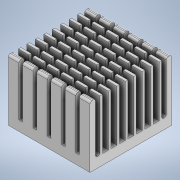
# Autodesk Inventor part: Część2
Saved by Autodesk Inventor 2022 (Build 260153000, 153)
## iProperties
Created: 2022-09-09
Part Number: Część2
Material: Ogólny
Document SubType Name: Modeling
Designer: kosak
Density: 1 g/cm^3
Appearance: Domyślna
Author: kosak
Autodesk Inventor part; units mm, degrees
ref_plane "YZ Plane" through (0, 0, 0) normal (1, 0, 0) x (0, 1, 0)
ref_plane "XZ Plane" through (0, 0, 0) normal (0, 1, 0) x (-1, 0, 0)
ref_plane "XY Plane" through (0, 0, 0) normal (0, 0, 1) x (1, 0, 0)
sketch "Szkic1" plane through (0, 0, 0) normal (0, 1, 0) x (-1, 0, 0)
  line L0 (0, 0) -> (40, 0)
  line L1 (40, 0) -> (40, -40)
  line L2 (40, -40) -> (0, -40)
  line L3 (0, -40) -> (0, 0)
  dimension "d0" = 40
  dimension "d1" = 40
  constraints: 8 end point, 2 parallel, 1 horizontal, 1 perpendicular
  measures "d0" distance of L1.end L2.end
  measures "d1" distance of L0.end L1.end
extrude "Wyciągnięcie proste1" add sketch "Szkic1" along normal blind 5
sketch "Szkic2" plane through (0, 5, 0) normal (0, 1, 0) x (1, 0, 0)
  line L0 (0, 20) -> (-40, 20)
  line L1 (-20, 0) -> (-20, 40)
  line L2 (0, 40) -> (-5.2, 40)
  line L3 (-5.2, 40) -> (-5.2, 37.35)
  line L4 (-5.2, 37.35) -> (0, 37.35)
  line L5 (0, 37.35) -> (0, 40)
  line L6 (-40, 37.35) -> (-40, 40)
  line L7 (-34.8, 37.35) -> (-40, 37.35)
  line L8 (-34.8, 40) -> (-34.8, 37.35)
  line L9 (-40, 40) -> (-34.8, 40)
  line L10 (-12.16, 40) -> (-12.16, 37.35)
  line L11 (-6.96, 40) -> (-12.16, 40)
  line L12 (-12.16, 37.35) -> (-6.96, 37.35)
  line L13 (-6.96, 37.35) -> (-6.96, 40)
  line L14 (-19.12, 40) -> (-19.12, 37.35)
  line L15 (-13.92, 40) -> (-19.12, 40)
  line L16 (-19.12, 37.35) -> (-13.92, 37.35)
  line L17 (-13.92, 37.35) -> (-13.92, 40)
  line L18 (-26.08, 40) -> (-26.08, 37.35)
  line L19 (-20.88, 40) -> (-26.08, 40)
  line L20 (-26.08, 37.35) -> (-20.88, 37.35)
  line L21 (-20.88, 37.35) -> (-20.88, 40)
  line L22 (-33.04, 40) -> (-33.04, 37.35)
  line L23 (-27.84, 40) -> (-33.04, 40)
  line L24 (-33.04, 37.35) -> (-27.84, 37.35)
  line L25 (-27.84, 37.35) -> (-27.84, 40)
  line L26 (-40, 40) -> (-40, 37.35)
  line L27 (-34.8, 40) -> (-40, 40)
  line L28 (-40, 37.35) -> (-34.8, 37.35)
  line L29 (-34.8, 37.35) -> (-34.8, 40)
  line L30 (-34.8, 2.65) -> (-40, 2.65)
  line L31 (-40, 2.65) -> (-40, 0)
  line L32 (-40, 0) -> (-34.8, 0)
  line L33 (-5.2, 0) -> (-5.2, 2.65)
  line L34 (-5.2, 2.65) -> (0, 2.65)
  line L35 (0, 2.65) -> (0, 0)
  line L36 (0, 0) -> (-5.2, 0)
  line L37 (-12.16, 0) -> (-12.16, 2.65)
  line L38 (-6.96, 0) -> (-12.16, 0)
  line L39 (-12.16, 2.65) -> (-6.96, 2.65)
  line L40 (-6.96, 2.65) -> (-6.96, 0)
  line L41 (-19.12, 0) -> (-19.12, 2.65)
  line L42 (-13.92, 0) -> (-19.12, 0)
  line L43 (-19.12, 2.65) -> (-13.92, 2.65)
  line L44 (-13.92, 2.65) -> (-13.92, 0)
  line L45 (-26.08, 0) -> (-26.08, 2.65)
  line L46 (-20.88, 0) -> (-26.08, 0)
  line L47 (-26.08, 2.65) -> (-20.88, 2.65)
  line L48 (-20.88, 2.65) -> (-20.88, 0)
  line L49 (-33.04, 0) -> (-33.04, 2.65)
  line L50 (-27.84, 0) -> (-33.04, 0)
  line L51 (-33.04, 2.65) -> (-27.84, 2.65)
  line L52 (-27.84, 2.65) -> (-27.84, 0)
  line L53 (-34.8, 2.65) -> (-34.8, 0)
  line L54 (-2.6, 37.35) -> (-2.6, 35.1)
  line L55 (0, 0) -> (0, 40) projected
  line L56 (0, 35.1) -> (-5.2, 35.1)
  line L57 (-5.2, 35.1) -> (-5.2, 33.86)
  line L58 (-5.2, 33.86) -> (0, 33.86)
  line L59 (0, 33.86) -> (0, 35.1)
  line L60 (-6.96, 35.1) -> (-12.16, 35.1)
  line L61 (-12.16, 33.86) -> (-6.96, 33.86)
  line L62 (-12.16, 35.1) -> (-12.16, 33.86)
  line L63 (-6.96, 33.86) -> (-6.96, 35.1)
  line L64 (-13.92, 35.1) -> (-19.12, 35.1)
  line L65 (-19.12, 33.86) -> (-13.92, 33.86)
  line L66 (-19.12, 35.1) -> (-19.12, 33.86)
  line L67 (-13.92, 33.86) -> (-13.92, 35.1)
  line L68 (-20.88, 35.1) -> (-26.08, 35.1)
  line L69 (-26.08, 33.86) -> (-20.88, 33.86)
  line L70 (-26.08, 35.1) -> (-26.08, 33.86)
  line L71 (-20.88, 33.86) -> (-20.88, 35.1)
  line L72 (-27.84, 35.1) -> (-33.04, 35.1)
  line L73 (-33.04, 33.86) -> (-27.84, 33.86)
  line L74 (-33.04, 35.1) -> (-33.04, 33.86)
  line L75 (-27.84, 33.86) -> (-27.84, 35.1)
  line L76 (-34.8, 35.1) -> (-40, 35.1)
  line L77 (-40, 33.86) -> (-34.8, 33.86)
  line L78 (-40, 35.1) -> (-40, 33.86)
  line L79 (-34.8, 33.86) -> (-34.8, 35.1)
  line L80 (0, 4.9) -> (-5.2, 4.9)
  line L81 (-5.2, 4.9) -> (-5.2, 6.14)
  line L82 (-5.2, 6.14) -> (0, 6.14)
  line L83 (0, 30.963) -> (-5.2, 30.963)
  line L84 (-5.2, 29.723) -> (0, 29.723)
  line L85 (-5.2, 30.963) -> (-5.2, 29.723)
  line L86 (0, 29.723) -> (0, 30.963)
  line L87 (0, 26.826) -> (-5.2, 26.826)
  line L88 (-5.2, 25.586) -> (0, 25.586)
  line L89 (-5.2, 26.826) -> (-5.2, 25.586)
  line L90 (0, 25.586) -> (0, 26.826)
  line L91 (0, 22.689) -> (-5.2, 22.689)
  line L92 (-5.2, 21.449) -> (0, 21.449)
  line L93 (-5.2, 22.689) -> (-5.2, 21.449)
  line L94 (0, 21.449) -> (0, 22.689)
  line L95 (0, 18.552) -> (-5.2, 18.552)
  line L96 (-5.2, 17.312) -> (0, 17.312)
  line L97 (-5.2, 18.552) -> (-5.2, 17.312)
  line L98 (0, 17.312) -> (0, 18.552)
  line L99 (0, 14.415) -> (-5.2, 14.415)
  line L100 (-5.2, 13.175) -> (0, 13.175)
  line L101 (-5.2, 14.415) -> (-5.2, 13.175)
  line L102 (0, 13.175) -> (0, 14.415)
  line L103 (0, 10.278) -> (-5.2, 10.278)
  line L104 (-5.2, 9.038) -> (0, 9.038)
  line L105 (-5.2, 10.278) -> (-5.2, 9.038)
  line L106 (0, 9.038) -> (0, 10.278)
  line L107 (0, 6.141) -> (-5.2, 6.141)
  line L108 (-5.2, 4.901) -> (0, 4.901)
  line L109 (-5.2, 6.141) -> (-5.2, 4.901)
  line L110 (0, 4.901) -> (0, 6.141)
  line L111 (-6.96, 30.963) -> (-12.16, 30.963)
  line L112 (-6.96, 29.723) -> (-6.96, 30.963)
  line L113 (-12.16, 29.723) -> (-6.96, 29.723)
  line L114 (-12.16, 30.963) -> (-12.16, 29.723)
  line L115 (-13.92, 30.963) -> (-19.12, 30.963)
  line L116 (-19.12, 29.723) -> (-13.92, 29.723)
  line L117 (-13.92, 29.723) -> (-13.92, 30.963)
  line L118 (-20.88, 29.723) -> (-20.88, 30.963)
  line L119 (-20.88, 30.963) -> (-26.08, 30.963)
  line L120 (-26.08, 29.723) -> (-20.88, 29.723)
  line L121 (-26.08, 30.963) -> (-26.08, 29.723)
  line L122 (-27.84, 29.723) -> (-27.84, 30.963)
  line L123 (-27.84, 30.963) -> (-33.04, 30.963)
  line L124 (-33.04, 29.723) -> (-27.84, 29.723)
  line L125 (-33.04, 30.963) -> (-33.04, 29.723)
  line L126 (-34.8, 29.723) -> (-34.8, 30.963)
  line L127 (-34.8, 30.963) -> (-40, 30.963)
  line L128 (-40, 29.723) -> (-34.8, 29.723)
  line L129 (-40, 30.963) -> (-40, 29.723)
  line L130 (-6.96, 26.826) -> (-12.16, 26.826)
  line L131 (-6.96, 25.586) -> (-6.96, 26.826)
  line L132 (-12.16, 25.586) -> (-6.96, 25.586)
  line L133 (-12.16, 26.826) -> (-12.16, 25.586)
  line L134 (-13.92, 26.826) -> (-19.12, 26.826)
  line L135 (-19.12, 25.586) -> (-13.92, 25.586)
  line L136 (-13.92, 25.586) -> (-13.92, 26.826)
  line L137 (-20.88, 25.586) -> (-20.88, 26.826)
  line L138 (-20.88, 26.826) -> (-26.08, 26.826)
  line L139 (-26.08, 25.586) -> (-20.88, 25.586)
  line L140 (-26.08, 26.826) -> (-26.08, 25.586)
  line L141 (-27.84, 25.586) -> (-27.84, 26.826)
  line L142 (-27.84, 26.826) -> (-33.04, 26.826)
  line L143 (-33.04, 25.586) -> (-27.84, 25.586)
  line L144 (-33.04, 26.826) -> (-33.04, 25.586)
  line L145 (-34.8, 25.586) -> (-34.8, 26.826)
  line L146 (-34.8, 26.826) -> (-40, 26.826)
  line L147 (-40, 25.586) -> (-34.8, 25.586)
  line L148 (-40, 26.826) -> (-40, 25.586)
  line L149 (-6.96, 22.689) -> (-12.16, 22.689)
  line L150 (-6.96, 21.449) -> (-6.96, 22.689)
  line L151 (-12.16, 21.449) -> (-6.96, 21.449)
  line L152 (-12.16, 22.689) -> (-12.16, 21.449)
  line L153 (-13.92, 22.689) -> (-19.12, 22.689)
  line L154 (-19.12, 21.449) -> (-13.92, 21.449)
  line L155 (-13.92, 21.449) -> (-13.92, 22.689)
  line L156 (-20.88, 21.449) -> (-20.88, 22.689)
  line L157 (-20.88, 22.689) -> (-26.08, 22.689)
  line L158 (-26.08, 21.449) -> (-20.88, 21.449)
  line L159 (-26.08, 22.689) -> (-26.08, 21.449)
  line L160 (-27.84, 21.449) -> (-27.84, 22.689)
  line L161 (-27.84, 22.689) -> (-33.04, 22.689)
  line L162 (-33.04, 21.449) -> (-27.84, 21.449)
  line L163 (-33.04, 22.689) -> (-33.04, 21.449)
  line L164 (-34.8, 21.449) -> (-34.8, 22.689)
  line L165 (-34.8, 22.689) -> (-40, 22.689)
  line L166 (-40, 21.449) -> (-34.8, 21.449)
  line L167 (-40, 22.689) -> (-40, 21.449)
  line L168 (-6.96, 18.552) -> (-12.16, 18.552)
  line L169 (-6.96, 17.312) -> (-6.96, 18.552)
  line L170 (-12.16, 17.312) -> (-6.96, 17.312)
  line L171 (-12.16, 18.552) -> (-12.16, 17.312)
  line L172 (-13.92, 18.552) -> (-19.12, 18.552)
  line L173 (-19.12, 17.312) -> (-13.92, 17.312)
  line L174 (-13.92, 17.312) -> (-13.92, 18.552)
  line L175 (-20.88, 17.312) -> (-20.88, 18.552)
  line L176 (-20.88, 18.552) -> (-26.08, 18.552)
  line L177 (-26.08, 17.312) -> (-20.88, 17.312)
  line L178 (-26.08, 18.552) -> (-26.08, 17.312)
  line L179 (-27.84, 17.312) -> (-27.84, 18.552)
  line L180 (-27.84, 18.552) -> (-33.04, 18.552)
  line L181 (-33.04, 17.312) -> (-27.84, 17.312)
  line L182 (-33.04, 18.552) -> (-33.04, 17.312)
  line L183 (-34.8, 17.312) -> (-34.8, 18.552)
  line L184 (-34.8, 18.552) -> (-40, 18.552)
  line L185 (-40, 17.312) -> (-34.8, 17.312)
  line L186 (-40, 18.552) -> (-40, 17.312)
  line L187 (-6.96, 14.415) -> (-12.16, 14.415)
  line L188 (-6.96, 13.175) -> (-6.96, 14.415)
  line L189 (-12.16, 13.175) -> (-6.96, 13.175)
  line L190 (-12.16, 14.415) -> (-12.16, 13.175)
  line L191 (-13.92, 14.415) -> (-19.12, 14.415)
  line L192 (-19.12, 13.175) -> (-13.92, 13.175)
  line L193 (-13.92, 13.175) -> (-13.92, 14.415)
  line L194 (-20.88, 13.175) -> (-20.88, 14.415)
  line L195 (-20.88, 14.415) -> (-26.08, 14.415)
  line L196 (-26.08, 13.175) -> (-20.88, 13.175)
  line L197 (-26.08, 14.415) -> (-26.08, 13.175)
  line L198 (-27.84, 13.175) -> (-27.84, 14.415)
  line L199 (-27.84, 14.415) -> (-33.04, 14.415)
  line L200 (-33.04, 13.175) -> (-27.84, 13.175)
  line L201 (-33.04, 14.415) -> (-33.04, 13.175)
  line L202 (-34.8, 13.175) -> (-34.8, 14.415)
  line L203 (-34.8, 14.415) -> (-40, 14.415)
  line L204 (-40, 13.175) -> (-34.8, 13.175)
  line L205 (-40, 14.415) -> (-40, 13.175)
  line L206 (-6.96, 10.278) -> (-12.16, 10.278)
  line L207 (-6.96, 9.038) -> (-6.96, 10.278)
  line L208 (-12.16, 9.038) -> (-6.96, 9.038)
  line L209 (-12.16, 10.278) -> (-12.16, 9.038)
  line L210 (-13.92, 10.278) -> (-19.12, 10.278)
  line L211 (-19.12, 9.038) -> (-13.92, 9.038)
  line L212 (-13.92, 9.038) -> (-13.92, 10.278)
  line L213 (-20.88, 9.038) -> (-20.88, 10.278)
  line L214 (-20.88, 10.278) -> (-26.08, 10.278)
  line L215 (-26.08, 9.038) -> (-20.88, 9.038)
  line L216 (-26.08, 10.278) -> (-26.08, 9.038)
  line L217 (-27.84, 9.038) -> (-27.84, 10.278)
  line L218 (-27.84, 10.278) -> (-33.04, 10.278)
  line L219 (-33.04, 9.038) -> (-27.84, 9.038)
  line L220 (-33.04, 10.278) -> (-33.04, 9.038)
  line L221 (-34.8, 9.038) -> (-34.8, 10.278)
  line L222 (-34.8, 10.278) -> (-40, 10.278)
  line L223 (-40, 9.038) -> (-34.8, 9.038)
  line L224 (-40, 10.278) -> (-40, 9.038)
  line L225 (-6.96, 6.141) -> (-12.16, 6.141)
  line L226 (-6.96, 4.901) -> (-6.96, 6.141)
  line L227 (-12.16, 4.901) -> (-6.96, 4.901)
  line L228 (-12.16, 6.141) -> (-12.16, 4.901)
  line L229 (-13.92, 6.141) -> (-19.12, 6.141)
  line L230 (-19.12, 4.901) -> (-13.92, 4.901)
  line L231 (-13.92, 4.901) -> (-13.92, 6.141)
  line L232 (-20.88, 4.901) -> (-20.88, 6.141)
  line L233 (-20.88, 6.141) -> (-26.08, 6.141)
  line L234 (-26.08, 4.901) -> (-20.88, 4.901)
  line L235 (-26.08, 6.141) -> (-26.08, 4.901)
  line L236 (-27.84, 4.901) -> (-27.84, 6.141)
  line L237 (-27.84, 6.141) -> (-33.04, 6.141)
  line L238 (-33.04, 4.901) -> (-27.84, 4.901)
  line L239 (-33.04, 6.141) -> (-33.04, 4.901)
  line L240 (-34.8, 4.901) -> (-34.8, 6.141)
  line L241 (-34.8, 6.141) -> (-40, 6.141)
  line L242 (-40, 4.901) -> (-34.8, 4.901)
  line L243 (-40, 6.141) -> (-40, 4.901)
  line L244 (-19.12, 30.963) -> (-19.12, 29.723)
  line L245 (-19.12, 26.826) -> (-19.12, 25.586)
  line L246 (-19.12, 22.689) -> (-19.12, 21.449)
  line L247 (-19.12, 18.552) -> (-19.12, 17.312)
  line L248 (-19.12, 14.415) -> (-19.12, 13.175)
  line L249 (-19.12, 10.278) -> (-19.12, 9.038)
  line L250 (-19.12, 6.141) -> (-19.12, 4.901)
  dimension "d8" = 6.96
  dimension "d13" = 2.25
  dimension "d14" = 1.24
  dimension "d17" = 6.96
  dimension "d24" = 4.137
  dimension "d31" = 4.137
  dimension "d40" = 4.137
  constraints: 500 end point, 32 symmetric about line, 28 vertical alignment, 16 parallel, 14 collinear, 4 vertical, 3 horizontal, 1 midpoint, 1 perpendicular, 376 other
  measures "d8" distance of L3.start L10.start
  measures "d13" distance of L54.start L54.end
  measures "d14" distance of L57.end L56.end
  measures "d17" distance of L56.start L60.start
  measures "d24" distance of L56.start L83.start
  measures "d31" distance of L60.start L111.start
  measures "d40" distance of L64.end L244.start
extrude "Wyciągnięcie proste2" add sketch "Szkic2" along normal blind 25 contours L5 L4 L3 L2 | L35 L36 L33 L34 | L55 L80 L81 L82 | L55 L104 L105 L103 | L55 L100 L101 L99 | L55 L96 L97 L95 | L55 L92 L93 L91 | L55 L88 L89 L87 | L55 L84 L85 L83 | L55 L58 L57 L56 | L6 L9 L8 L7 | L11 L13 L12 L10 | L15 L17 L16 L14 | L19 L21 L20 L18 | L23 L25 L24 L22 | L53 L32 L31 L30 | L37 L39 L40 L38 | L41 L43 L44 L42 | L45 L47 L48 L46 | L49 L51 L52 L50 | L63 L61 L62 L60 | L67 L65 L66 L64 | L71 L69 L70 L68 | L75 L73 L74 L72 | L79 L77 L78 L76 | L112 L113 L114 L111 | L117 L116 L244 L115 | L120 L121 L119 L118 | L124 L125 L123 L122 | L128 L129 L127 L126 | L131 L132 L133 L130 | L136 L135 L245 L134 | L139 L140 L138 L137 | L143 L144 L142 L141 | L147 L148 L146 L145 | L150 L151 L152 L149 | L155 L154 L246 L153 | L158 L159 L157 L156 | L162 L163 L161 L160 | L166 L167 L165 L164 | L169 L170 L171 L168 | L174 L173 L247 L172 | L177 L178 L176 L175 | L181 L182 L180 L179 | L185 L186 L184 L183 | L188 L189 L190 L187 | L193 L192 L248 L191 | L196 L197 L195 L194 | L200 L201 L199 L198 | L204 L205 L203 L202 | L207 L208 L209 L206 | L212 L211 L249 L210 | L215 L216 L214 L213 | L219 L220 L218 L217 | L223 L224 L222 L221 | L226 L227 L228 L225 | L231 L230 L250 L229 | L234 L235 L233 L232 | L238 L239 L237 L236 | L242 L243 L241 L240
fillet "Zaokrąglenie1" radius 1 2 edges at (-2.6, 5, -4.901) (-2.6, 5, -2.65)
pattern_linear "Szyk prostokątny1" count 6 spacing 6.96 along (-1, 0, 0) of "Zaokrąglenie1"
fillet "Zaokrąglenie2" radius 1 2 edges at (-2.6, 5, -35.1) (-2.6, 5, -37.35)
fillet "Zaokrąglenie3" radius 1 2 edges at (-2.6, 30, -2.65) (-2.6, 30, 0)
pattern_linear "Szyk prostokątny2" count 6 spacing 6.96 along (-1, 0, 0) of "Zaokrąglenie3"
fillet "Zaokrąglenie4" radius 1 2 edges at (-2.6, 30, -40) (-2.6, 30, -37.35)
pattern_linear "Szyk prostokątny3" count 6 spacing 6.96 along (-1, 0, 0) of "Zaokrąglenie4"
